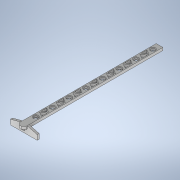
# Autodesk Inventor part: pEndpice-corner
Saved by Autodesk Inventor 2020.1 (Build 241239000, 239)
## iProperties
Created: 2019-08-25
Part Number: pEndpice-corner
Material: Generic
Document SubType Name: Modeling
Designer: niels
Density: 1 g/cm^3
Appearance: Default
Author: niels
Autodesk Inventor part; units mm, degrees
ref_plane "YZ Plane" through (0, 0, 0) normal (1, 0, 0) x (0, 1, 0)
sketch "Sketch1" plane through (0, 0, 0) normal (0, 1, 0) x (-1, 0, 0)
  line L0 (0, 0) -> (10, 0)
  line L1 (10, 0) -> (10, -200)
  line L2 (10, -200) -> (0, -200)
  line L3 (0, -200) -> (0, 0)
  dimension "d0" = 10
  dimension "d1" = 200
  constraints: 8 end point, 2 parallel, 1 horizontal, 1 perpendicular
  measures "d0" distance of L1.end L2.end
  measures "d1" distance of L0.end L1.end
extrude "ExtrusionBase" add sketch "Sketch1" along normal blind 4
sketch "Sketch2" plane through (0, 4, 0) normal (0, 1, 0) x (1, 0, 0)
  circle A0 centre (-5, 15) radius 3.05
  line L0 (0, 0) -> (0, 200) projected
  line L1 (-10, 0) -> (0, 0) projected
  dimension "d5" = 6.1
  dimension "d6" = 5
  dimension "d7" = 15
  constraints: 1 centre point
  measures "d5" diameter of A0
  measures "d6" distance from line of A0.centre L0
  measures "d7" distance from line of L1 A0.centre
extrude "ExtrusionHole" cut sketch "Sketch2" against normal up to surface (4 mm away)
fillet "FilletHole" radius 0.8 2 edges at (-8.05, 4, -15) (-8.05, 0, -15)
sketch "Sketch3" plane through (0, 4, 0) normal (0, 1, 0) x (1, 0, 0)
  line L0 (-1.5, 28.0915) -> (-1.5, 20.0085)
  line L1 (-1.5, 20.0085) -> (-8.5, 24.05)
  line L2 (-8.5, 24.05) -> (-1.5, 28.0915)
  line L3 (-1.5, 30.5741) -> (-8.5, 26.5326)
  line L4 (-8.5, 26.5326) -> (-8.5, 34.6155)
  line L5 (-8.5, 34.6155) -> (-1.5, 30.5741)
  line L6 (0, 0) -> (0, 200) projected
  line L7 (-10, 200) -> (-10, 0) projected
  circle A0 centre (-5, 15) radius 3.05 projected
  point P0 (-3.8333, 24.05)
  point P1 (-6.1667, 30.5741)
  dimension "d14" = 1.5
  dimension "d15" = 1.5
  dimension "d16" = 1.5
  dimension "d17" = 1.5
  dimension "d18" = 2.15
  dimension "d19" = 9.05
  constraints: 12 end point, 2 parallel, 14 other
  measures "d14" distance between parallel lines of L0 L6
  measures "d15" distance from line of L7 L1.end
  measures "d16" distance between parallel lines of L7 L4
  measures "d17" distance from line of L6 L3.start
  measures "d18" distance between parallel lines of L3 L2
  measures "d19" vertical distance of point (-3.833, 24.05) A0.centre
extrude "ExtrusionBaseCutout" cut sketch "Sketch3" against normal up to surface (4 mm away) contours L0 L1 L2 | L3 L4 L5
pattern_linear "Rectangular PatternHoles" count 8 spacing 25 along (0, 0, -1) of "FilletHole", "ExtrusionHole"
pattern_linear "Rectangular PatternBaseCutout" count 7 spacing 25 along (0, 0, -1) of "ExtrusionBaseCutout"
sketch "Sketch5" plane through (-10, 0, 0) normal (0, 0, 1) x (1, 0, 0)
  line L0 (0, 0) -> (0, 4) projected
  line L1 (10, 0) -> (7.5, -4.3301)
  line L2 (7.5, -4.3301) -> (2.5, -4.3301)
  line L3 (2.5, -4.3301) -> (0, 0)
  line L4 (1.7321, 0) -> (3.366, 2.8301)
  line L5 (3.366, 2.8301) -> (6.634, 2.8301)
  line L6 (6.634, 2.8301) -> (8.2679, 0)
  line L7 (8.2679, 0) -> (6.634, -2.8301)
  line L8 (6.634, -2.8301) -> (3.366, -2.8301)
  line L9 (3.366, -2.8301) -> (1.7321, 0)
  line L10 (10, 0) -> (10, 4) projected
  line L11 (10, 0) -> (0, 0)
  line L12 (0, 0) -> (0, 4)
  line L13 (0, 4) -> (10, 4)
  line L14 (10, 4) -> (10, 0)
  line L15 (8.2679, 0) -> (1.7321, 0)
  line L16 (1.5, 0) -> (8.5, 0) projected
  line L17 (1.7321, 0) -> (8.2679, 0)
  point P0 (5, 0)
  point P1 (5, 0)
  point P2 (1.7321, 0)
  dimension "d28" = 1.5
  constraints: 30 end point, 2 collinear, 2 parallel, 1 coincident, 1 horizontal, 1 perpendicular, 19 other
  measures "d28" distance between parallel lines of L3 L9
extrude "Extrusion Horizontal" add sketch "Sketch5" along normal blind 3 contours L11 L9 L8 L7 L1 L2 L3 | L0 L13 L10 L11 L6 L5 L4 | L4 L5 L6 L11
sketch "Sketch6" plane through (-10, 0, 3) normal (0, 0, 1) x (1, 0, 0)
  line L0 (7.5, -4.3301) -> (10, 0) projected
  line L1 (0, 0) -> (0, 4) projected
  line L2 (10, 0) -> (0, 0)
  line L3 (0, 0) -> (0, 4)
  line L4 (0, 4) -> (10, 4)
  line L5 (10, 4) -> (10, 0)
  constraints: 8 end point, 2 parallel, 1 horizontal, 1 perpendicular
extrude "ExtrusionHorizontalSupport" add sketch "Sketch6" along normal blind 5
ref_plane "Work Plane1" through (-5, -8.6603, 0) normal (-1, 0, 0) x (0, 0, -1)
sketch "Sketch7" plane through (-5, -8.6603, 0) normal (-1, 0, 0) x (0, 0, -1)
  line L0 (-3, -8.6603) -> (-8, -8.6603) projected
  line L1 (-3, -4.3301) -> (-3, -8.6603) projected
  line L2 (-8, -8.6603) -> (-3, -4.3301)
  line L3 (-5.7087, -8.6603) -> (-3, -6.3144)
  line L4 (-8, -8.6603) -> (-5.7087, -8.6603)
  line L5 (-3, -6.3144) -> (-3, -4.3301)
  point P0 (0, -8.6603)
  dimension "d33" = 1.5
  constraints: 8 end point, 2 point on line, 1 collinear, 1 parallel
  measures "d33" distance between parallel lines of L2 L3
extrude "ExtrusionHorizontalRib" add sketch "Sketch7" along normal mid plane 3 contours L0 L2 L1 L3
chamfer "ChamferHorizontalSupport" distance 3.5 angle 45 2 edges at (-10, 2, 8) (0, 2, 8)
sketch "Sketch8" plane through (-7.5, -4.3301, 0) normal (0, -1, 0) x (1, 0, 0)
  line L0 (0, 0) -> (0, 3) projected
  line L1 (5, 0) -> (5, 3) projected
  line L2 (0, 3) -> (5, 3)
  line L3 (5, 3) -> (5, 0)
  line L4 (5, 0) -> (0, 0)
  line L5 (0, 0) -> (0, 3)
  point P0 (7.5, 0)
  constraints: 8 end point, 2 parallel, 1 horizontal, 1 perpendicular
extrude "ExtrusionHorizontalExtended" add sketch "Sketch8" along normal blind 3
sketch "Sketch13" plane through (0, 0, 0) normal (0, -1, 0) x (1, 0, 0)
  line L0 (-9.5, -10.293) -> (-9.5, 0.3869) construction
  line L1 (-9.5, 0.3869) -> (-0.5, 0.3869) construction
  line L2 (-0.5, 0.3869) -> (-0.5, -10.293) construction
  line L3 (-0.5, -10.293) -> (-9.5, -10.293) construction
  line L4 (0, 0) -> (0, -200) projected
  spline S0 degree 2 poles (-7.3287, -8.068) (-6.5159, -8.068) (-5.9488, -8.4501) knots 0 0 0 1 1 1
  spline S1 degree 2 poles (-5.9488, -8.4501) (-5.3271, -8.8686) (-5.3271, -9.5479) knots 0 0 0 1 1 1
  spline S2 degree 2 poles (-5.3271, -9.5479) (-5.3271, -10.0574) (-5.6971, -10.4153) knots 0 0 0 1 1 1
  line L5 (-5.6971, -10.4153) -> (-5.3271, -10.667)
  spline S3 degree 2 poles (-5.3271, -10.667) (-5.2331, -10.7307) (-5.2331, -10.8247) knots 0 0 0 1 1 1
  spline S4 degree 2 poles (-5.2331, -10.8247) (-5.2331, -11.0006) (-5.3908, -11.0006) knots 0 0 0 1 1 1
  spline S5 degree 2 poles (-5.3908, -11.0006) (-5.4272, -11.0006) (-5.4848, -10.9702) knots 0 0 0 1 1 1
  line L6 (-5.4848, -10.9702) -> (-5.961, -10.6579)
  spline S6 degree 2 poles (-5.961, -10.6579) (-6.5402, -11.0521) (-7.3287, -11.0521) knots 0 0 0 1 1 1
  spline S7 degree 2 poles (-7.3287, -11.0521) (-8.1353, -11.0521) (-8.7297, -10.6761) knots 0 0 0 1 1 1
  spline S8 degree 2 poles (-8.7297, -10.6761) (-9.3726, -10.2636) (-9.3726, -9.6147) knots 0 0 0 1 1 1
  spline S9 degree 2 poles (-9.3726, -9.6147) (-9.3726, -9.1264) (-9.0481, -8.7655) knots 0 0 0 1 1 1
  line L7 (-9.0481, -8.7655) -> (-9.403, -8.532)
  spline S10 degree 2 poles (-9.403, -8.532) (-9.5, -8.4683) (-9.5, -8.3713) knots 0 0 0 1 1 1
  spline S11 degree 2 poles (-9.5, -8.3713) (-9.5, -8.2015) (-9.3271, -8.2075) knots 0 0 0 1 1 1
  spline S12 degree 2 poles (-9.3271, -8.2075) (-9.2817, -8.2075) (-9.2453, -8.2318) knots 0 0 0 1 1 1
  line L8 (-9.2453, -8.2318) -> (-8.7934, -8.5229)
  spline S13 degree 2 poles (-8.7934, -8.5229) (-8.1899, -8.068) (-7.3287, -8.068) knots 0 0 0 1 1 1
  spline S14 degree 2 poles (-7.3317, -8.4228) (-7.9867, -8.4228) (-8.4629, -8.714) knots 0 0 0 1 1 1
  line L9 (-8.4629, -8.714) -> (-5.9943, -10.2424)
  spline S15 degree 2 poles (-5.9943, -10.2424) (-5.688, -9.9543) (-5.688, -9.5479) knots 0 0 0 1 1 1
  spline S16 degree 2 poles (-5.688, -9.5479) (-5.688, -9.0021) (-6.1975, -8.6958) knots 0 0 0 1 1 1
  spline S17 degree 2 poles (-6.1975, -8.6958) (-6.6585, -8.4228) (-7.3317, -8.4228) knots 0 0 0 1 1 1
  spline S18 degree 2 poles (-8.7388, -8.9445) (-9.0057, -9.2295) (-9.0057, -9.6116) knots 0 0 0 1 1 1
  spline S19 degree 2 poles (-9.0057, -9.6116) (-9.0057, -10.1332) (-8.4719, -10.4304) knots 0 0 0 1 1 1
  spline S20 degree 2 poles (-8.4719, -10.4304) (-8.008, -10.6912) (-7.3287, -10.6912) knots 0 0 0 1 1 1
  spline S21 degree 2 poles (-7.3287, -10.6912) (-6.7373, -10.6912) (-6.2976, -10.4608) knots 0 0 0 1 1 1
  line L10 (-6.2976, -10.4608) -> (-8.7388, -8.9445)
  spline S22 degree 2 poles (-6.7737, -4.7018) (-6.1459, -4.7018) (-5.3271, -5.3933) (-5.3271, -5.9513) knots 0 0 0 1 2 2 2
  spline S23 degree 2 poles (-5.3271, -5.9513) (-5.3271, -6.6457) (-5.8154, -7.0248) knots 0 0 0 1 1 1
  spline S24 degree 2 poles (-5.8154, -7.0248) (-6.243, -7.3493) (-6.9162, -7.3493) knots 0 0 0 1 1 1
  spline S25 degree 2 poles (-6.9162, -7.3493) (-7.271, -7.3493) (-7.6198, -7.2492) knots 0 0 0 1 1 1
  spline S26 degree 2 poles (-7.6198, -7.2492) (-8.1717, -7.0946) (-8.5599, -6.7792) knots 0 0 0 1 1 1
  spline S27 degree 2 poles (-8.5599, -6.7792) (-8.9784, -6.4486) (-9.3423, -5.833) knots 0 0 0 1 1 1
  spline S28 degree 2 poles (-9.3423, -5.833) (-9.3726, -5.7875) (-9.3726, -5.742) knots 0 0 0 1 1 1
  spline S29 degree 2 poles (-9.3726, -5.742) (-9.3726, -5.6723) (-9.2574, -5.5722) (-9.1816, -5.5722) knots 0 0 0 1 2 2 2
  spline S30 degree 2 poles (-9.1816, -5.5722) (-9.0815, -5.5722) (-9.0299, -5.6601) knots 0 0 0 1 1 1
  spline S31 degree 2 poles (-9.0299, -5.6601) (-8.4962, -6.5426) (-7.7532, -6.8156) knots 0 0 0 1 1 1
  spline S32 degree 2 poles (-7.7532, -6.8156) (-7.6774, -6.8429) (-7.6259, -6.855) knots 0 0 0 1 1 1
  spline S33 degree 2 poles (-7.6259, -6.855) (-8.0444, -6.5366) (-8.0444, -5.9786) knots 0 0 0 1 1 1
  spline S34 degree 2 poles (-8.0444, -5.9786) (-8.0444, -5.3751) (-7.3772, -4.7018) (-6.7737, -4.7018) knots 0 0 0 1 2 2 2
  spline S35 degree 2 poles (-6.7737, -5.0567) (-7.1497, -5.0567) (-7.6774, -5.6025) (-7.6774, -5.9786) knots 0 0 0 1 2 2 2
  spline S36 degree 2 poles (-7.6774, -5.9786) (-7.6774, -6.3849) (-7.0982, -6.949) (-6.6857, -6.949) knots 0 0 0 1 2 2 2
  spline S37 degree 2 poles (-6.6857, -6.949) (-6.2672, -6.949) (-5.688, -6.3637) (-5.688, -5.9513) knots 0 0 0 1 2 2 2
  spline S38 degree 2 poles (-5.688, -5.9513) (-5.688, -5.557) (-6.0246, -5.2993) knots 0 0 0 1 1 1
  spline S39 degree 2 poles (-6.0246, -5.2993) (-6.337, -5.0567) (-6.7737, -5.0567) knots 0 0 0 1 1 1
  spline S40 degree 2 poles (-5.6365, -3.2943) (-5.4083, -3.2943) (-5.2358, -3.3607) knots 0 0 0 1 1 1
  spline S41 degree 2 poles (-5.2358, -3.3607) (-5.0978, -3.4111) (-4.8696, -3.5623) knots 0 0 0 1 1 1
  spline S42 degree 2 poles (-4.8696, -3.5623) (-4.798, -3.6075) (-4.798, -3.6579) knots 0 0 0 1 1 1
  spline S43 degree 2 poles (-4.798, -3.6579) (-4.798, -3.7295) (-4.8935, -3.7295) knots 0 0 0 1 1 1
  spline S44 degree 2 poles (-4.8935, -3.7295) (-4.9492, -3.7295) (-5.0049, -3.695) knots 0 0 0 1 1 1
  spline S45 degree 2 poles (-5.0049, -3.695) (-5.2092, -3.5677) (-5.3658, -3.5677) knots 0 0 0 1 1 1
  spline S46 degree 2 poles (-5.3658, -3.5677) (-5.3976, -3.5677) (-5.4215, -3.573) knots 0 0 0 1 1 1
  spline S47 degree 2 poles (-5.4215, -3.573) (-5.525, -3.8012) (-5.6975, -3.8012) knots 0 0 0 1 1 1
  spline S48 degree 2 poles (-5.6975, -3.8012) (-5.7267, -3.8012) (-5.7638, -3.7959) knots 0 0 0 1 1 1
  spline S49 degree 2 poles (-5.7638, -3.7959) (-5.9814, -3.7561) (-5.9814, -3.573) knots 0 0 0 1 1 1
  spline S50 degree 2 poles (-5.9814, -3.573) (-5.9814, -3.4615) (-5.793, -3.2943) (-5.6365, -3.2943) knots 0 0 0 1 2 2 2
  spline S51 degree 2 poles (-7.3317, -0.0468) (-6.519, -0.0468) (-5.9488, -0.3592) knots 0 0 0 1 1 1
  spline S52 degree 2 poles (-5.9488, -0.3592) (-5.3271, -0.7018) (-5.3271, -1.2477) knots 0 0 0 1 1 1
  spline S53 degree 2 poles (-5.3271, -1.2477) (-5.3271, -1.7936) (-5.9488, -2.1363) knots 0 0 0 1 1 1
  spline S54 degree 2 poles (-5.9488, -2.1363) (-6.522, -2.4486) (-7.3317, -2.4486) knots 0 0 0 1 1 1
  spline S55 degree 2 poles (-7.3317, -2.4486) (-8.1323, -2.4486) (-8.7115, -2.1302) knots 0 0 0 1 1 1
  spline S56 degree 2 poles (-8.7115, -2.1302) (-9.3393, -1.7875) (-9.3393, -1.2477) knots 0 0 0 1 1 1
  spline S57 degree 2 poles (-9.3393, -1.2477) (-9.3393, -0.7018) (-8.7115, -0.3592) knots 0 0 0 1 1 1
  spline S58 degree 2 poles (-8.7115, -0.3592) (-8.1384, -0.0468) (-7.3317, -0.0468) knots 0 0 0 1 1 1
  spline S59 degree 2 poles (-7.3347, -0.3956) (-7.9928, -0.3956) (-8.4629, -0.6169) knots 0 0 0 1 1 1
  spline S60 degree 2 poles (-8.4629, -0.6169) (-8.9723, -0.8535) (-8.9723, -1.2477) knots 0 0 0 1 1 1
  spline S61 degree 2 poles (-8.9723, -1.2477) (-8.9723, -1.6359) (-8.4568, -1.8724) knots 0 0 0 1 1 1
  spline S62 degree 2 poles (-8.4568, -1.8724) (-7.9867, -2.0938) (-7.3317, -2.0938) knots 0 0 0 1 1 1
  spline S63 degree 2 poles (-7.3317, -2.0938) (-6.6736, -2.0938) (-6.2036, -1.8724) knots 0 0 0 1 1 1
  spline S64 degree 2 poles (-6.2036, -1.8724) (-5.688, -1.6359) (-5.688, -1.2477) knots 0 0 0 1 1 1
  spline S65 degree 2 poles (-5.688, -1.2477) (-5.688, -0.8595) (-6.2036, -0.6169) knots 0 0 0 1 1 1
  spline S66 degree 2 poles (-6.2036, -0.6169) (-6.6797, -0.3956) (-7.3347, -0.3956) knots 0 0 0 1 1 1
  line L11 (-1.8532, -7.3787) -> (-2.1835, -7.041)
  line L12 (-2.1835, -7.041) -> (-2.1835, -10.0318)
  line L13 (-2.1835, -10.0318) -> (-1.8532, -9.6867)
  line L14 (-1.8532, -9.6867) -> (-1.4414, -9.6867)
  line L15 (-1.4414, -9.6867) -> (-2.3653, -10.5772)
  line L16 (-2.3653, -10.5772) -> (-2.3764, -10.5772)
  line L17 (-2.3764, -10.5772) -> (-3.3041, -9.6867)
  line L18 (-3.3041, -9.6867) -> (-2.8922, -9.6867)
  line L19 (-2.8922, -9.6867) -> (-2.5545, -10.0355)
  line L20 (-2.5545, -10.0355) -> (-2.5545, -7.0373)
  line L21 (-2.5545, -7.0373) -> (-2.8922, -7.3787)
  line L22 (-2.8922, -7.3787) -> (-3.3041, -7.3787)
  line L23 (-3.3041, -7.3787) -> (-2.3764, -6.4882)
  line L24 (-2.3764, -6.4882) -> (-2.3653, -6.4882)
  line L25 (-2.3653, -6.4882) -> (-1.4414, -7.3787)
  line L26 (-1.4414, -7.3787) -> (-1.8532, -7.3787)
  line L27 (-0.709, -3.598) -> (-0.709, -5.8087)
  spline S67 degree 2 poles (-0.709, -5.8087) (-1.076, -5.7087) (-1.4338, -5.6116) knots 0 0 0 1 1 1
  spline S68 degree 2 poles (-1.4338, -5.6116) (-1.9221, -5.4539) (-2.2799, -5.1749) knots 0 0 0 1 1 1
  spline S69 degree 2 poles (-2.2799, -5.1749) (-2.756, -4.805) (-3.123, -4.1529) knots 0 0 0 1 1 1
  spline S70 degree 2 poles (-3.123, -4.1529) (-3.3413, -3.7587) (-3.7265, -3.7587) knots 0 0 0 1 1 1
  spline S71 degree 2 poles (-3.7265, -3.7587) (-3.963, -3.7587) (-4.1328, -3.9285) knots 0 0 0 1 1 1
  spline S72 degree 2 poles (-4.1328, -3.9285) (-4.3057, -4.1135) (-4.3057, -4.4138) knots 0 0 0 1 1 1
  spline S73 degree 2 poles (-4.3057, -4.4138) (-4.3057, -4.7473) (-4.2086, -4.9323) knots 0 0 0 1 1 1
  spline S74 degree 2 poles (-4.2086, -4.9323) (-4.0843, -5.1476) (-3.7719, -5.275) knots 0 0 0 1 1 1
  spline S75 degree 2 poles (-3.7719, -5.275) (-3.6628, -5.3205) (-3.6628, -5.4266) knots 0 0 0 1 1 1
  spline S76 degree 2 poles (-3.6628, -5.4266) (-3.6628, -5.6056) (-3.8387, -5.6056) knots 0 0 0 1 1 1
  spline S77 degree 2 poles (-3.8387, -5.6056) (-3.872, -5.6056) (-3.9114, -5.5874) knots 0 0 0 1 1 1
  spline S78 degree 2 poles (-3.9114, -5.5874) (-4.6726, -5.275) (-4.6726, -4.438) knots 0 0 0 1 1 1
  spline S79 degree 2 poles (-4.6726, -4.438) (-4.6726, -3.9467) (-4.3936, -3.6495) knots 0 0 0 1 1 1
  spline S80 degree 2 poles (-4.3936, -3.6495) (-4.1389, -3.3766) (-3.7568, -3.3766) knots 0 0 0 1 1 1
  spline S81 degree 2 poles (-3.7568, -3.3766) (-3.1594, -3.3766) (-2.8106, -3.9862) knots 0 0 0 1 1 1
  spline S82 degree 2 poles (-2.8106, -3.9862) (-2.4042, -4.6988) (-1.8826, -5.0203) knots 0 0 0 1 1 1
  spline S83 degree 2 poles (-1.8826, -5.0203) (-1.6218, -5.1749) (-1.0699, -5.3266) knots 0 0 0 1 1 1
  line L28 (-1.0699, -5.3266) -> (-1.0699, -3.598)
  spline S84 degree 2 poles (-1.0699, -3.598) (-1.0699, -3.416) (-0.891, -3.416) knots 0 0 0 1 1 1
  spline S85 degree 2 poles (-0.891, -3.416) (-0.709, -3.416) (-0.709, -3.598) knots 0 0 0 1 1 1
  spline S86 degree 2 poles (-2.0191, -0.1924) (-1.4459, -0.1924) (-1.079, -0.4653) knots 0 0 0 1 1 1
  spline S87 degree 2 poles (-1.079, -0.4653) (-0.6848, -0.7655) (-0.6453, -1.3296) knots 0 0 0 1 1 1
  spline S88 degree 2 poles (-0.6453, -1.3296) (-0.612, -1.7693) (-0.894, -2.1181) knots 0 0 0 1 1 1
  spline S89 degree 2 poles (-0.894, -2.1181) (-1.1548, -2.4395) (-1.6036, -2.5942) knots 0 0 0 1 1 1
  spline S90 degree 2 poles (-1.6036, -2.5942) (-1.637, -2.6063) (-1.6734, -2.6063) knots 0 0 0 1 1 1
  spline S91 degree 2 poles (-1.6734, -2.6063) (-1.8462, -2.6063) (-1.8462, -2.4213) knots 0 0 0 1 1 1
  spline S92 degree 2 poles (-1.8462, -2.4213) (-1.8462, -2.3061) (-1.7249, -2.2636) knots 0 0 0 1 1 1
  spline S93 degree 2 poles (-1.7249, -2.2636) (-1.3944, -2.1423) (-1.1973, -1.9149) knots 0 0 0 1 1 1
  spline S94 degree 2 poles (-1.1973, -1.9149) (-0.982, -1.6662) (-1.0062, -1.3539) knots 0 0 0 1 1 1
  spline S95 degree 2 poles (-1.0062, -1.3539) (-1.0365, -0.9475) (-1.3307, -0.7322) knots 0 0 0 1 1 1
  spline S96 degree 2 poles (-1.3307, -0.7322) (-1.5976, -0.5411) (-2.0191, -0.5411) knots 0 0 0 1 1 1
  spline S97 degree 2 poles (-2.0191, -0.5411) (-2.4255, -0.5411) (-3.0229, -1.0749) (-3.0229, -1.4297) knots 0 0 0 1 2 2 2
  spline S98 degree 2 poles (-3.0229, -1.4297) (-3.0229, -1.9028) (-2.7864, -2.206) knots 0 0 0 1 1 1
  spline S99 degree 2 poles (-2.7864, -2.206) (-2.6893, -2.3334) (-2.6893, -2.391) knots 0 0 0 1 1 1
  spline S100 degree 2 poles (-2.6893, -2.391) (-2.6893, -2.5305) (-2.8379, -2.5305) knots 0 0 0 1 1 1
  line L29 (-2.8379, -2.5305) -> (-4.6332, -2.5305)
  line L30 (-4.6332, -2.5305) -> (-4.6332, -0.6806)
  spline S101 degree 2 poles (-4.6332, -0.6806) (-4.6332, -0.4926) (-4.4543, -0.4926) knots 0 0 0 1 1 1
  spline S102 degree 2 poles (-4.4543, -0.4926) (-4.2723, -0.4926) (-4.2723, -0.6776) knots 0 0 0 1 1 1
  line L31 (-4.2723, -0.6776) -> (-4.2723, -2.1757)
  line L32 (-4.2723, -2.1757) -> (-3.2049, -2.1757)
  spline S103 degree 2 poles (-3.2049, -2.1757) (-3.2564, -2.0726) (-3.3019, -1.9604) knots 0 0 0 1 1 1
  spline S104 degree 2 poles (-3.3019, -1.9604) (-3.3838, -1.742) (-3.3838, -1.4266) knots 0 0 0 1 1 1
  spline S105 degree 2 poles (-3.3838, -1.4266) (-3.3838, -0.9475) (-2.5771, -0.1924) (-2.0191, -0.1924) knots 0 0 0 1 2 2 2
  dimension "d73" = 9
  dimension "d75" = 0.5
  constraints: 2 other
  measures "d73" distance of L2.end L0.start
  measures "d75" distance between parallel lines of L2 L4
emboss "EmbossText" sketch "Sketch13" operation cut depth 1 direction (0, 1, 0)
sketch "Sketch15" plane through (-10, 0, 0) normal (0, 0, -1) x (-1, 0, 0)
  line L0 (-1.7321, 0) -> (0, 0) construction
  line L1 (0, 0) -> (-10, 0) construction
  line L2 (-10, 0) -> (-10, 3.9052) construction
  line L3 (-10, 3.9052) -> (0, 3.9052) construction
  line L4 (0, 3.9052) -> (0, 0) construction
  line L5 (-3.5, 0) -> (-6.5, 0) construction
  line L6 (-5, 0) -> (-25, 0)
  line L7 (-25, 0) -> (-25, -7.3301)
  line L8 (-25, -7.3301) -> (-5, -7.3301)
  line L9 (-5, -7.3301) -> (-5, 0) construction
  line L10 (-7.5, -7.3301) -> (-2.5, -7.3301) construction
  line L11 (-6.5, 0) -> (-10, 0) construction
  line L12 (-10, 0) -> (-5.1213, -7.3301)
  dimension "d80" = 15
  constraints: 18 end point, 4 parallel, 2 horizontal, 2 perpendicular, 1 collinear, 1 midpoint, 1 point on line
  measures "d80" distance from line of L7 L11.end
extrude "Extrusion12" add sketch "Sketch15" against normal up to surface (3 mm away)
ref_plane "Work Plane4" through (-5, 0, -200) normal (-1, 0, 0) x (0, 0, 1)
mirror "Mirror1" about plane through (-5, 0, -200) normal (-1, 0, 0) of "Extrusion12"
sketch "Sketch17" plane through (-10, 0, 3) normal (0, 0, 1) x (1, 0, 0)
  line L0 (10, 0) -> (10, 4) projected
  line L1 (10, 0) -> (25, 0) projected
  line L2 (10, 4) -> (25, 0)
  line L3 (25, 0) -> (10, 0)
  line L4 (10, 0) -> (10, 4)
  line L5 (0, 0) -> (0, 4) projected
  line L6 (0, 4.0002) -> (0, 0)
  line L7 (-15, 0) -> (-15, -7.3301) projected
  line L8 (0, 0) -> (-15, 0)
  line L9 (-15, 0) -> (0, 4.0002)
  constraints: 12 end point, 2 collinear, 2 perpendicular
extrude "Extrusion13" add sketch "Sketch17" against normal up to surface (3 mm away)
equation "\"d6\" = 0.5 * d0"
equation "\"d27\" = d24"
equation "\"d75\" = -0.5 * d73 + 0.5 * d0"
equation "\"d24\" = 25"
body "Solid1"
